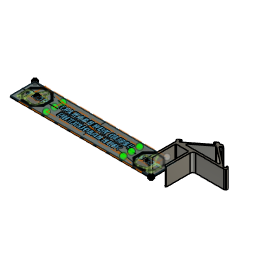
dishwasher sign (Autodesk Fusion 360 design; units mm, degrees)
Autodesk Fusion 360 part; units mm, degrees
sketch "Sketch1" plane through (0, 0, 0) normal (0, 0, 1) x (1, 0, 0) in component "holder"
  line L0 (0, 0) -> (0, 35)
  line L1 (0, 35) -> (18.4, 35)
  line L2 (18.4, 35) -> (18.4, 0)
  line L3 (-3, 0) -> (-3, 38)
  line L4 (-3, 38) -> (21.4, 38)
  line L5 (21.4, 38) -> (21.4, 0)
  line L6 (0, 0) -> (-3, 0)
  line L7 (18.4, 0) -> (21.4, 0)
  line L8 (31.7, 38) -> (31.7, 65) construction
  line L9 (66.4, 38) -> (31.7, 65)
  line L10 (31.7, 65) -> (-3, 38)
  line L11 (-3, 38) -> (66.4, 38)
  line L12 (5.7408, 41) -> (57.6592, 41)
  line L13 (57.6592, 41) -> (31.7, 61.1988)
  line L14 (31.7, 61.1988) -> (5.7408, 41)
  line L15 (28.2996, 62.3542) -> (26.8565, 64.2089)
  line L16 (31.7, 65) -> (29.3357, 68.0385)
  line L17 (29.3357, 68.0385) -> (24.7515, 64.4716)
  line L18 (24.7515, 64.4716) -> (25.6727, 63.2877)
  line L19 (25.6727, 63.2877) -> (26.8565, 64.2089)
  line L20 (14.35, 51.5) -> (5.8308, 62.4488) construction
  line L21 (-5.3643, 41.0385) -> (-0.7801, 44.6055)
  line L22 (-3, 38) -> (-5.3643, 41.0385)
  line L23 (0.4004, 40.6458) -> (-1.0428, 42.5005)
  line L24 (0.1411, 43.4217) -> (-1.0428, 42.5005)
  line L25 (-0.7801, 44.6055) -> (0.1411, 43.4217)
  line L26 (31.7, 65) -> (34.0643, 68.0385)
  line L27 (34.0643, 68.0385) -> (38.6485, 64.4716)
  line L28 (38.6485, 64.4716) -> (37.7273, 63.2877)
  line L29 (37.7273, 63.2877) -> (36.5435, 64.2089)
  line L30 (35.1004, 62.3542) -> (36.5435, 64.2089)
  line L31 (62.9996, 40.6458) -> (64.4428, 42.5005)
  line L32 (63.2589, 43.4217) -> (64.4428, 42.5005)
  line L33 (64.1801, 44.6055) -> (63.2589, 43.4217)
  line L34 (68.7643, 41.0385) -> (64.1801, 44.6055)
  line L35 (66.4, 38) -> (68.7643, 41.0385)
  dimension "d8" = 35
  dimension "d9" = 18.4
  dimension "d10" = 35
  dimension "d12" = 45
  dimension "d19" = 2.35
  dimension "d20" = 3.85
  dimension "d21" = 17.675
  dimension "d22" = 1.5
  dimension "d31" = 30
  constraint coincident L0.start L6.start
  constraint vertical L0
  constraint perpendicular L0 L1
  constraint perpendicular L1 L2
  constraint perpendicular L3 L6
  constraint coincident L4 L8.start
  constraint perpendicular L4 L8
  constraint equal L9 L10
  constraint perpendicular L3 L11
  constraint coincident L10 L15.start
  constraint perpendicular L10 L15
  constraint perpendicular L10 L16
  constraint perpendicular L16 L17
  constraint perpendicular L17 L18
  constraint parallel L17 L19
  constraint midpoint L10 L20.start
  constraint perpendicular L10 L20
  constraint symmetric L8.end L20 L3.end
  constraint symmetric L15.start L20 L23.start
  constraint symmetric L15.end L20 L23.end
  constraint symmetric L16.end L20 L21.start
  constraint symmetric L17.end L20 L21.end
  constraint symmetric L18.end L20 L24.start
  constraint symmetric L9.end L8 L10.start
  constraint symmetric L8 L15.start L30.start
  constraint symmetric L8 L15.end L29.end
  constraint symmetric L8 L16.end L26.end
  constraint symmetric L8 L17.end L27.end
  constraint symmetric L8 L18.end L28.end
  constraint symmetric L8 L21.start L34.start
  constraint symmetric L8 L21.end L33.start
  constraint symmetric L8 L3.end L9.start
  constraint symmetric L8 L23.start L31.start
  constraint symmetric L8 L23.end L31.end
  constraint symmetric L8 L24.start L32.start
  measures "d8" distance of L0.start L0.end
  measures "d9" distance of L0.end L1.end
  measures "d10" distance of L1.end L2.end
  measures "d12" distance of L4.end L9.start
  measures "d19" distance of L15.start L15.end
  measures "d20" distance of L8.end L16.end
  measures "d21" distance of L15 L20
  measures "d22" distance of L15 L18
  measures "d31" distance of L1 L8.end
extrude "Extrude1" add sketch "Sketch1" along normal blind 25 makes body 1 in component "holder"
fillet "Fillet1" radius 4 1 edges at (21.4, 38, 12.5) on bodies 1 in component "holder"
fillet "Fillet2" radius 2 7 edges at (-3, 38, 12.5) (-5.3643, 41.0385, 12.5) (66.4, 38, 12.5) (68.7643, 41.0385, 12.5) (31.7, 65, 12.5) (34.0643, 68.0385, 12.5) (29.3357, 68.0385, 12.5) on bodies 1 in component "holder"
fillet "Fillet3" radius 1 5 edges at (18.4, 35, 12.5) (31.7, 61.1988, 12.5) (5.7408, 41, 12.5) (57.6592, 41, 12.5) (0, 35, 12.5) on bodies 1 in component "holder"
sketch "Sketch1 (2)" plane through (0, 0, 0) normal (0, 0, 1) x (1, 0, 0) in component "stop_sign"
  line L0 (0, 0) -> (-200, 0)
  line L1 (-200, 0) -> (-200, 34.8)
  line L2 (-200, 34.8) -> (0, 34.8)
  line L3 (0, 34.8) -> (0, 0)
  dimension "d32" = 200
  dimension "d33" = 34.8
  constraint horizontal L0
  constraint vertical L1
  constraint horizontal L2
  constraint vertical L3
  constraint coincident L0.start L3.end
  measures "d32" distance of L0.start L0.end
  measures "d33" distance of L0.start L2.end
extrude "Extrude1'" add sketch "Sketch1 (2)" along normal blind 1.825 separate body makes body 2 in component "stop_sign"
sketch "Sketch2" plane through (0, 0, 1.825) normal (0, 0, 1) x (-1, 0, 0) in component "stop_sign"
  line L0 (0, -34.8) -> (200, -34.8)
  line L1 (200, -34.8) -> (200, 0)
  line L2 (200, 0) -> (0, 0)
  line L3 (0, 0) -> (0, -34.8)
  line L4 (165.2, -11.4353) -> (165.2, -23.3647)
  line L5 (165.2, -23.3647) -> (173.6353, -31.8)
  line L6 (173.6353, -31.8) -> (185.5647, -31.8)
  line L7 (185.5647, -31.8) -> (194, -23.3647)
  line L8 (194, -23.3647) -> (194, -11.4353)
  line L9 (194, -11.4353) -> (185.5647, -3)
  line L10 (185.5647, -3) -> (173.6353, -3)
  line L11 (173.6353, -3) -> (165.2, -11.4353)
  line L12 (200, -17.4) -> (0, -17.4) construction
  line L13 (186.674, 1.0426) -> (13.326, 1.0426) construction
  line L14 (13.326, 1.0426) -> (13.326, -35.8426) construction
  line L15 (13.326, -35.8426) -> (186.674, -35.8426) construction
  line L16 (186.674, -35.8426) -> (186.674, 1.0426) construction
  line L17 (186.0617, -33) -> (195.2, -23.8617)
  line L18 (195.2, -23.8617) -> (195.2, -10.9383)
  line L19 (195.2, -10.9383) -> (186.0617, -1.8)
  line L20 (186.0617, -1.8) -> (173.1383, -1.8)
  line L21 (173.1383, -1.8) -> (164, -10.9383)
  line L22 (164, -10.9383) -> (164, -23.8617)
  line L23 (164, -23.8617) -> (173.1383, -33)
  line L24 (173.1383, -33) -> (186.0617, -33)
  line L25 (187.3312, -11.7516) -> (171.8688, -11.7516) construction
  line L26 (171.8688, -11.7516) -> (171.8688, -23.0484) construction
  line L27 (171.8688, -23.0484) -> (187.3312, -23.0484) construction
  line L28 (187.3312, -23.0484) -> (187.3312, -11.7516) construction
  line L29 (187.3312, -23.0484) -> (171.8688, -11.7516) construction
  line L30 (200, -34.8) -> (0, 0) construction
  line L31 (186.674, -35.8426) -> (13.326, 1.0426) construction
  line L32 (100, -34.8) -> (100, 0) construction
  line L33 (34.8, -23.3647) -> (26.3647, -31.8)
  line L34 (4.8, -10.9383) -> (13.9383, -1.8)
  line L35 (6, -11.4353) -> (14.4353, -3)
  line L36 (26.8617, -1.8) -> (36, -10.9383)
  line L37 (26.3647, -31.8) -> (14.4353, -31.8)
  line L38 (4.8, -23.8617) -> (4.8, -10.9383)
  line L39 (34.8, -11.4353) -> (34.8, -23.3647)
  line L40 (36, -10.9383) -> (36, -23.8617)
  line L41 (6, -23.3647) -> (6, -11.4353)
  line L42 (26.3647, -3) -> (34.8, -11.4353)
  line L43 (14.4353, -3) -> (26.3647, -3)
  line L44 (36, -23.8617) -> (26.8617, -33)
  line L45 (14.4353, -31.8) -> (6, -23.3647)
  line L46 (26.8617, -33) -> (13.9383, -33)
  line L47 (13.9383, -1.8) -> (26.8617, -1.8)
  line L48 (13.9383, -33) -> (4.8, -23.8617)
  line L49 (29.5065, -11.8018) -> (11.2935, -11.8018) construction
  line L50 (11.2935, -11.8018) -> (11.2935, -22.9982) construction
  line L51 (11.2935, -22.9982) -> (29.5065, -22.9982) construction
  line L52 (29.5065, -22.9982) -> (29.5065, -11.8018) construction
  line L53 (11.2935, -22.9982) -> (29.5065, -11.8018) construction
  point P0 (179.6, -17.4)
  point P1 (20.4, -17.4)
  point P2 (13.326, -35.8426)
  dimension "d38" = 3
  dimension "d39" = 3
  dimension "d40" = 6
  dimension "d42" = 7
  dimension "d50" = 1.2
  dimension "d51" = 7
  dimension "d57" = 7
  text T0 "DISHWASHER IN USE\nPUT CUPS IN SINK" font "Arial" height 7 bold align centre middle in box 173.348 x 36.8852 at (186.674, 1.0426) x (-1, 0) y (0, -1) spacing 1 kerned
  text T1 "STOP" font "Arial" height 7 bold align centre middle in box 15.4623 x 11.2968 at (187.3312, -11.7516) x (-1, 0) y (0, -1) spacing 1 kerned
  text T2 "STOP" font "Arial" height 7 bold align centre middle in box 18.2129 x 11.1965 at (29.5065, -11.8018) x (-1, 0) y (0, -1) spacing 1 kerned
  constraint horizontal L6
  constraint midpoint L1 L12.start
  constraint midpoint L3 L12.end
  constraint coincident L12
  constraint vertical L16
  constraint coincident L27.end
  constraint coincident L25.end
  constraint midpoint P0 L29
  constraint coincident L0.end L1.start
  constraint coincident L2.end L3.start
  constraint coincident L15.end
  constraint coincident L13.end
  constraint midpoint L30 L31
  constraint midpoint L0 L32.start
  constraint midpoint L2 L32.end
  constraint symmetric L4.start L32 L39.start
  constraint symmetric L4.end L32 L33.start
  constraint symmetric L5.end L32 L33.end
  constraint symmetric L6.end L32 L37.end
  constraint symmetric L7.end L32 L41.start
  constraint symmetric L8.end L32 L35.start
  constraint symmetric L9.end L32 L35.end
  constraint symmetric L10.end L32 L42.start
  constraint symmetric P0 L32 P1
  constraint symmetric L17.start L32 L46.end
  constraint symmetric L17.end L32 L38.start
  constraint symmetric L18.end L32 L34.start
  constraint symmetric L19.end L32 L34.end
  constraint symmetric L20.end L32 L36.start
  constraint symmetric L21.end L32 L36.end
  constraint symmetric L22.end L32 L40.end
  constraint symmetric L23.end L32 L44.end
  constraint symmetric L15.end L32 P2
  constraint coincident L50.end
  constraint coincident L49.start
  constraint midpoint P1 L53
  measures "d38" distance of L0 L6
  measures "d39" distance of L2 L10
  measures "d40" distance of L1 L8
extrude "Extrude2" add sketch "Sketch2" sketch "Sketch2" along normal blind 0.6 contours L17 L18 L19 L20 L21 L22 L23 L24 | L34 L36 L38 L40 L44 L46 L47 L48 of sketch 2 text T1 T0 T2 bodies 2 in component "stop_sign"
sketch "Sketch1 (3)" plane through (0, 0, 0) normal (0, 0, 1) x (1, 0, 0) in component "go_sign"
  line L0 (0, 0) -> (-200, 0)
  line L1 (-200, 0) -> (-200, 34.8)
  line L2 (-200, 34.8) -> (0, 34.8)
  line L3 (0, 34.8) -> (0, 0)
  dimension "d32_1" = 200
  dimension "d33_1" = 34.8
  constraint horizontal L0
  constraint vertical L1
  constraint horizontal L2
  constraint vertical L3
  constraint coincident L0.start L3.end
  measures "d32_1" distance of L0.start L0.end
  measures "d33_1" distance of L0.start L2.end
extrude "Extrude1''" add sketch "Sketch1 (3)" along normal blind 1.825 separate body makes body 3 in component "go_sign"
sketch "Sketch2 (2)" plane through (0, 0, 1.825) normal (0, 0, 1) x (-1, 0, 0) in component "go_sign"
  line L0 (0, -34.8) -> (200, -34.8)
  line L1 (200, -34.8) -> (200, 0)
  line L2 (200, 0) -> (0, 0)
  line L3 (0, 0) -> (0, -34.8)
  line L4 (200, -17.4) -> (0, -17.4) construction
  line L5 (154.5846, -5.7854) -> (45.4154, -5.7854) construction
  line L6 (45.4154, -5.7854) -> (45.4154, -29.0146) construction
  line L7 (45.4154, -29.0146) -> (154.5846, -29.0146) construction
  line L8 (154.5846, -29.0146) -> (154.5846, -5.7854) construction
  line L9 (154.5846, -29.0146) -> (45.4154, -5.7854) construction
  line L10 (10.5033, -19.8023) -> (6.27, -19.8023)
  spline S0 degree 3 poles (6.27, -19.8023) (5.5686, -19.8023) (5, -19.2337) (5, -18.5323) knots 0 0 0 0 1 1 1 1
  line L11 (5, -18.5323) -> (5, -5.8323)
  spline S1 degree 3 poles (5, -5.8323) (5, -5.1309) (5.5686, -4.5623) (6.27, -4.5623) knots 0 0 0 0 1 1 1 1
  line L12 (6.27, -4.5623) -> (10.5033, -4.5623)
  spline S2 degree 3 poles (10.5033, -4.5623) (11.2047, -4.5623) (11.7733, -5.1309) (11.7733, -5.8323) knots 0 0 0 0 1 1 1 1
  line L13 (11.7733, -5.8323) -> (11.7733, -18.5323)
  spline S3 degree 3 poles (11.7733, -18.5323) (11.7733, -19.2337) (11.2047, -19.8023) (10.5033, -19.8023) knots 0 0 0 0 1 1 1 1
  spline S4 degree 3 poles (8.3867, -6.679) (7.6853, -6.679) (7.1167, -7.2475) (7.1167, -7.949) knots 0 0 0 0 1 1 1 1
  spline S5 degree 3 poles (7.1167, -7.949) (7.1167, -8.6504) (7.6853, -9.219) (8.3867, -9.219) knots 0 0 0 0 1 1 1 1
  spline S6 degree 3 poles (8.3867, -9.219) (9.0881, -9.219) (9.6567, -8.6504) (9.6567, -7.949) knots 0 0 0 0 1 1 1 1
  spline S7 degree 3 poles (9.6567, -7.949) (9.6567, -7.2475) (9.0881, -6.679) (8.3867, -6.679) knots 0 0 0 0 1 1 1 1
  spline S8 degree 3 poles (25.32, -27.3454) (25.32, -25.1009) (23.9458, -23.8419) (23.5591, -22.3423) knots 0 0 0 0 1 1 1 1
  line L14 (23.5591, -22.3423) -> (28.9419, -22.3423)
  spline S9 degree 3 poles (28.9419, -22.3423) (30.7092, -22.3423) (32.085, -20.8741) (32.0933, -19.2679) knots 0 0 0 0 1 1 1 1
  spline S10 degree 3 poles (32.0933, -19.2679) (32.0977, -18.3187) (31.694, -17.2968) (31.0646, -16.6646) knots 0 0 0 0 1 1 1 1
  line L15 (31.0646, -16.6646) -> (31.0588, -16.6588)
  spline S11 degree 3 poles (31.0588, -16.6588) (31.5793, -15.4239) (31.4947, -13.6935) (30.5663, -12.4535) knots 0 0 0 0 1 1 1 1
  spline S12 degree 3 poles (30.5663, -12.4535) (31.0256, -11.0833) (30.5626, -9.4) (29.6994, -8.4976) knots 0 0 0 0 1 1 1 1
  spline S13 degree 3 poles (29.6994, -8.4976) (29.9268, -7.5664) (29.8181, -6.7739) (29.3741, -6.1359) knots 0 0 0 0 1 1 1 1
  spline S14 degree 3 poles (29.3741, -6.1359) (28.294, -4.5841) (25.6172, -4.5623) (23.3536, -4.5623) knots 0 0 0 0 1 1 1 1
  line L16 (23.3536, -4.5623) -> (23.203, -4.5623)
  spline S15 degree 3 poles (23.203, -4.5623) (20.6478, -4.5632) (18.5566, -5.4936) (16.8763, -6.2411) knots 0 0 0 0 1 1 1 1
  spline S16 degree 3 poles (16.8763, -6.2411) (16.0319, -6.6168) (14.9279, -7.0818) (14.0902, -7.0972) knots 0 0 0 0 1 1 1 1
  spline S17 degree 3 poles (14.0902, -7.0972) (13.7441, -7.1036) (13.4667, -7.386) (13.4667, -7.7321) knots 0 0 0 0 1 1 1 1
  line L17 (13.4667, -7.7321) -> (13.4667, -19.0441)
  spline S18 degree 3 poles (13.4667, -19.0441) (13.4667, -19.2134) (13.5345, -19.3759) (13.6549, -19.495) knots 0 0 0 0 1 1 1 1
  spline S19 degree 3 poles (13.6549, -19.495) (15.7512, -21.5664) (16.6526, -23.7594) (18.3707, -25.4805) knots 0 0 0 0 1 1 1 1
  spline S20 degree 3 poles (18.3707, -25.4805) (19.1541, -26.2653) (19.439, -27.4509) (19.7144, -28.5974) knots 0 0 0 0 1 1 1 1
  spline S21 degree 3 poles (19.7144, -28.5974) (19.9498, -29.5764) (20.442, -31.6556) (21.51, -31.6556) knots 0 0 0 0 1 1 1 1
  spline S22 degree 3 poles (21.51, -31.6556) (22.78, -31.6556) (25.32, -31.2323) (25.32, -27.3454) knots 0 0 0 0 1 1 1 1
  line L18 (189.4819, -19.8023) -> (193.7152, -19.8023)
  spline S23 degree 3 poles (193.7152, -19.8023) (194.4166, -19.8023) (194.9852, -19.2337) (194.9852, -18.5323) knots 0 0 0 0 1 1 1 1
  line L19 (194.9852, -18.5323) -> (194.9852, -5.8323)
  spline S24 degree 3 poles (194.9852, -5.8323) (194.9852, -5.1309) (194.4166, -4.5623) (193.7152, -4.5623) knots 0 0 0 0 1 1 1 1
  line L20 (193.7152, -4.5623) -> (189.4819, -4.5623)
  spline S25 degree 3 poles (189.4819, -4.5623) (188.7805, -4.5623) (188.2119, -5.1309) (188.2119, -5.8323) knots 0 0 0 0 1 1 1 1
  line L21 (188.2119, -5.8323) -> (188.2119, -18.5323)
  spline S26 degree 3 poles (188.2119, -18.5323) (188.2119, -19.2337) (188.7805, -19.8023) (189.4819, -19.8023) knots 0 0 0 0 1 1 1 1
  spline S27 degree 3 poles (191.5985, -6.679) (192.3, -6.679) (192.8685, -7.2475) (192.8685, -7.949) knots 0 0 0 0 1 1 1 1
  spline S28 degree 3 poles (192.8685, -7.949) (192.8685, -8.6504) (192.3, -9.219) (191.5985, -9.219) knots 0 0 0 0 1 1 1 1
  spline S29 degree 3 poles (191.5985, -9.219) (190.8971, -9.219) (190.3285, -8.6504) (190.3285, -7.949) knots 0 0 0 0 1 1 1 1
  spline S30 degree 3 poles (190.3285, -7.949) (190.3285, -7.2475) (190.8971, -6.679) (191.5985, -6.679) knots 0 0 0 0 1 1 1 1
  spline S31 degree 3 poles (174.6652, -27.3454) (174.6652, -25.1009) (176.0395, -23.8419) (176.4261, -22.3423) knots 0 0 0 0 1 1 1 1
  line L22 (176.4261, -22.3423) -> (171.0433, -22.3423)
  spline S32 degree 3 poles (171.0433, -22.3423) (169.276, -22.3423) (167.9002, -20.8741) (167.8919, -19.2679) knots 0 0 0 0 1 1 1 1
  spline S33 degree 3 poles (167.8919, -19.2679) (167.8875, -18.3187) (168.2912, -17.2968) (168.9206, -16.6646) knots 0 0 0 0 1 1 1 1
  line L23 (168.9206, -16.6646) -> (168.9264, -16.6588)
  spline S34 degree 3 poles (168.9264, -16.6588) (168.4059, -15.4239) (168.4905, -13.6935) (169.4189, -12.4535) knots 0 0 0 0 1 1 1 1
  spline S35 degree 3 poles (169.4189, -12.4535) (168.9596, -11.0833) (169.4226, -9.4) (170.2858, -8.4976) knots 0 0 0 0 1 1 1 1
  spline S36 degree 3 poles (170.2858, -8.4976) (170.0584, -7.5664) (170.1671, -6.7739) (170.6112, -6.1359) knots 0 0 0 0 1 1 1 1
  spline S37 degree 3 poles (170.6112, -6.1359) (171.6912, -4.5841) (174.368, -4.5623) (176.6316, -4.5623) knots 0 0 0 0 1 1 1 1
  line L24 (176.6316, -4.5623) -> (176.7822, -4.5623)
  spline S38 degree 3 poles (176.7822, -4.5623) (179.3374, -4.5632) (181.4286, -5.4936) (183.1089, -6.2411) knots 0 0 0 0 1 1 1 1
  spline S39 degree 3 poles (183.1089, -6.2411) (183.9533, -6.6168) (185.0574, -7.0818) (185.895, -7.0972) knots 0 0 0 0 1 1 1 1
  spline S40 degree 3 poles (185.895, -7.0972) (186.2411, -7.1036) (186.5185, -7.386) (186.5185, -7.7321) knots 0 0 0 0 1 1 1 1
  line L25 (186.5185, -7.7321) -> (186.5185, -19.0441)
  spline S41 degree 3 poles (186.5185, -19.0441) (186.5185, -19.2134) (186.4507, -19.3759) (186.3303, -19.495) knots 0 0 0 0 1 1 1 1
  spline S42 degree 3 poles (186.3303, -19.495) (184.234, -21.5664) (183.3326, -23.7594) (181.6145, -25.4805) knots 0 0 0 0 1 1 1 1
  spline S43 degree 3 poles (181.6145, -25.4805) (180.8311, -26.2653) (180.5462, -27.4509) (180.2708, -28.5974) knots 0 0 0 0 1 1 1 1
  spline S44 degree 3 poles (180.2708, -28.5974) (180.0355, -29.5764) (179.5432, -31.6556) (178.4752, -31.6556) knots 0 0 0 0 1 1 1 1
  spline S45 degree 3 poles (178.4752, -31.6556) (177.2052, -31.6556) (174.6652, -31.2323) (174.6652, -27.3454) knots 0 0 0 0 1 1 1 1
  dimension "d42_1" = 7
  text T0 "PLEASE PUT CUPS\nIN DISHWASHER" font "Arial" height 7 bold align centre middle in box 109.1693 x 23.2292 at (154.5846, -5.7854) x (-1, 0) y (0, -1) spacing 1 kerned
  constraint midpoint L1 L4.start
  constraint midpoint L3 L4.end
  constraint coincident L4
  constraint vertical L8
  constraint coincident L7.end
  constraint coincident L5.end
  constraint midpoint L4 L9
extrude "Extrude3" add sketch "Sketch2 (2)" sketch "Sketch2 (2)" along normal blind 0.6 contours L10 S0 L11 S1 L12 S2 L13 S3 | S8 L14 S9 S10 L15 S11 S12 S13 S14 L16 S15 S16 S17 L17 S18 S19 S20 S21 S22 | L18 S23 L19 S24 L20 S25 L21 S26 | S31 L22 S32 S33 L23 S34 S35 S36 S37 L24 S38 S39 S40 L25 S41 S42 S43 S44 S45 of sketch 2 text T0 bodies 3 in component "go_sign"
fillet "Fillet4" radius 2 2 edges at (0, 0, 12.5) (18.4, 0, 12.5) on bodies 1 in component "holder"
chamfer "Chamfer1" distance 0.6 angle 45 20 edges at (-0.3212, 41.5732, 25) (26.2646, 63.7483, 25) (27.5781, 63.2815, 25) (14.35, 51.5, 25) (-0.4508, 42.9611, 25) (37.1354, 63.7483, 25) (35.8219, 63.2815, 25) (49.05, 51.5, 25) (63.7212, 41.5732, 25) (63.8508, 42.9611, 25) (63.8508, 42.9611, 0) (63.7212, 41.5732, 0) (49.05, 51.5, 0) (37.1354, 63.7483, 0) (35.8219, 63.2815, 0) (26.2646, 63.7483, 0) (27.5781, 63.2815, 0) (14.35, 51.5, 0) (-0.3212, 41.5732, 0) (-0.4508, 42.9611, 0) on bodies 1 in component "holder"
component "holder" placed x (1, 0, 0) y (0, 1, 0) z (0, 0, 1) at (0, 0, 0)
component "stop_sign" placed x (1, 0, 0) y (0, 1, 0) z (0, 0, 1) at (0, 0, 0)
component "go_sign" placed x (1, 0, 0) y (0, 1, 0) z (0, 0, 1) at (0, 0, 0)
equation "door_thickness = 18.4 mm"
equation "clip_height = 35 mm"
equation "sign_holder_height = 30 mm"
equation "sign_holder_overhang = 45 mm"
equation "thickness = 3 mm"
equation "d8 = clip_height"
equation "d9 = door_thickness"
equation "d10 = clip_height"
equation "d11 = -thickness"
equation "d12 = sign_holder_overhang"
equation "d14 = -thickness"
equation "sign_thickness = 2 mm"
equation "sign_height = 35 mm"
equation "width = 200 mm"
equation "d19 = sign_thickness + tolerance"
equation "d20 = sign_thickness + 0.5 * thickness + tolerance"
equation "d21 = sign_height / 2 + tolerance / 2"
equation "d22 = thickness / 2"
equation "d31 = sign_holder_height"
equation "d32 = width"
equation "d33 = sign_height - 0.2 mm"
equation "tolerance = 0.35 mm"
equation "d35 = sign_thickness - tolerance / 2"
equation "d39 = d38"
equation "d40 = 2 * d38"
equation "d32_1 = width"
equation "d33_1 = sign_height - 0.2 mm"
equation "d35_1 = sign_thickness - tolerance / 2"
